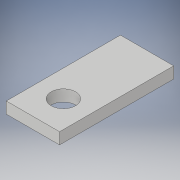
# Autodesk Inventor part: Picker Strip
Saved by Autodesk Inventor 2019.4 (Build 234330000, 330)
## iProperties
Created: 2021-01-07
Part Number: Picker Strip
Material: Generic
Document SubType Name: Modeling
Designer: caleb
Density: 1 g/cm^3
Appearance: Default
Author: caleb
Autodesk Inventor part; units mm, degrees
ref_plane "YZ Plane" through (0, 0, 0) normal (1, 0, 0) x (0, 1, 0)
ref_plane "XZ Plane" through (0, 0, 0) normal (0, 1, 0) x (-1, 0, 0)
ref_plane "XY Plane" through (0, 0, 0) normal (0, 0, 1) x (1, 0, 0)
sketch "Sketch1" plane through (0, 0, 0) normal (0, 1, 0) x (-1, 0, 0)
  line L0 (-3.5, 7.5) -> (3.5, 7.5)
  line L1 (3.5, 7.5) -> (3.5, -7.5)
  line L2 (3.5, -7.5) -> (-3.5, -7.5)
  line L3 (-3.5, -7.5) -> (-3.5, 7.5)
  line L4 (-3.5, 7.5) -> (3.5, -7.5) construction
  line L5 (3.5, 7.5) -> (-3.5, -7.5) construction
  circle A0 centre (0, 3.5) radius 1.6
  point P0 (0, 0)
  dimension "d0" = 15
  dimension "d1" = 7
  dimension "d2" = 3.2
  dimension "d3" = 4
  constraints: 12 end point, 2 midpoint, 2 parallel, 1 centre point, 1 horizontal, 1 perpendicular
  measures "d0" distance of L0.end L1.end
  measures "d1" distance of L0.start L0.end
  measures "d2" diameter of A0
  measures "d3" distance from line of L0 A0.centre
extrude "Extrusion1" add sketch "Sketch1" along normal blind 1.5
body "Solid1"
